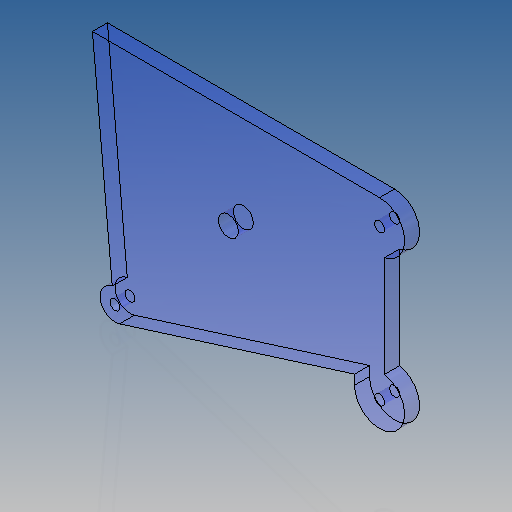
# Autodesk Inventor part: Protector
Saved by Autodesk Inventor 2017 (Build 210142000, 142)
## iProperties
Part Number: Protector
Material: Genérico
Document SubType Name: Modeling
Designer: Leo
Density: 1 g/cm^3
Appearance: Claro - Azul
Author: Leo
Autodesk Inventor part; units mm, degrees
ref_plane "YZ Plane" through (0, 0, 0) normal (1, 0, 0) x (0, 1, 0)
ref_plane "XZ Plane" through (0, 0, 0) normal (0, 1, 0) x (-1, 0, 0)
ref_plane "XY Plane" through (0, 0, 0) normal (0, 0, 1) x (1, 0, 0)
sketch "Boceto1" plane through (0, 0, 0) normal (0, 0, 1) x (1, 0, 0)
  circle A0 centre (22.1541, -50) radius 2 projected
  circle A1 centre (127.9669, -30) radius 2 projected
  circle A2 centre (127.9669, 30) radius 2 projected
  line L0 (21.0528, -44.1019) -> (13.1274, 40.1523)
  line L1 (13.1274, 40.1523) -> (127.9802, 40)
  arc A3 (129.9669, 20.202) -> (127.9802, 40) centre (127.9669, 30) ccw
  line L2 (129.9669, 20.202) -> (129.9669, -20.202)
  arc A4 (117.9669, -29.9867) -> (129.9669, -20.202) centre (127.9669, -30) ccw
  line L3 (117.9669, -29.9867) -> (117.9721, -26.1333)
  line L4 (117.9721, -26.1333) -> (23.9554, -55.7232)
  arc A5 (21.0528, -44.1019) -> (23.9554, -55.7232) centre (22.1541, -50) ccw
  circle A6 centre (67.5, 0) radius 40.0802 construction
  circle A7 centre (67.5, 0) radius 4 projected
  point P0 (0, 0)
  dimension "d0" = 10
  dimension "d1" = 8
  dimension "d4" = 6
  constraints: 10 end point, 6 point on circle, 5 tangent, 4 centre point, 4 concentric, 1 equal radius, 1 perpendicular
  measures "d0" radius of A3
  measures "d1" distance edge to line of A3 L2
  measures "d4" radius of A5
extrude "Extrusión1" add sketch "Boceto1" along normal blind 6
